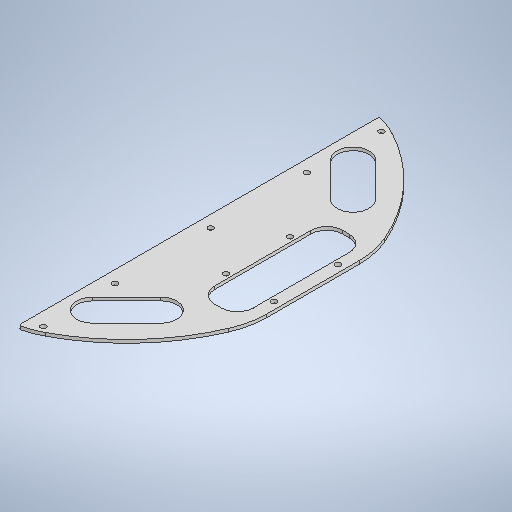
# Autodesk Inventor part: T2.0_frame-base2-extended-1
Saved by Autodesk Inventor 2025 (Build 290162000, 162)
## iProperties
Created: 2024-06-26
Part Number: T2.0_frame-base2-extended-1
Material: 一般
Document SubType Name: Sheet Metal
Designer: 8326d
Density: 1 g/cm^3
Sheet Metal Rule: Default_mm
Appearance: 既定
Author: 8326d
Autodesk Inventor part; units mm, degrees
ref_plane "YZ Plane" through (0, 0, 0) normal (1, 0, 0) x (0, 1, 0)
ref_plane "XZ Plane" through (0, 0, 0) normal (0, 1, 0) x (-1, 0, 0)
ref_plane "XY Plane" through (0, 0, 0) normal (0, 0, 1) x (1, 0, 0)
sketch "スケッチ1" plane through (0, 0, 0) normal (0, 1, 0) x (-1, 0, 0)
  circle A0 centre (0, 0) radius 122.5
  dimension "d0" = 245
  measures "d0" diameter of A0
extrude "プレート1" add sketch "スケッチ1" along normal blind 2
sketch "スケッチ2" plane through (0, 2, 0) normal (0, 1, 0) x (1, 0, 0)
  line L0 (85, -40) -> (109, -40)
  line L1 (109, -40) -> (109, 40)
  line L2 (109, 40) -> (85, 40)
  line L3 (85, 40) -> (85, -40)
  line L4 (85, -40) -> (109, 40) construction
  line L5 (109, -40) -> (85, 40) construction
  point P0 (0, 0)
  point P1 (97, 0)
  dimension "d2" = 24
  dimension "d3" = 85
  dimension "d6" = 80
  constraints: 12 end point, 2 midpoint, 2 parallel, 1 horizontal, 1 horizontal alignment, 1 perpendicular
  measures "d2" distance of L1.end L2.end
  measures "d3" distance from line of point (0, 0) L3
  measures "d6" distance of L0.end L1.end
extrude "押し出し1" cut sketch "スケッチ2" against normal through all
fillet "フィレット1" radius 10 4 edges at (109, 1, 40) (85, 1, 40) (85, 1, -40) (109, 1, -40)
sketch "スケッチ3" plane through (0, 2, 0) normal (0, 1, 0) x (1, 0, 0)
  line L0 (85, -30) -> (85, 30) projected
  line L1 (109, 30) -> (109, -30) projected
  line L2 (95, 40) -> (99, 40) projected
  line L3 (99, -40) -> (95, -40) projected
  line L4 (82, -20) -> (112, -20) construction
  line L5 (112, -20) -> (112, 20) construction
  line L6 (112, 20) -> (82, 20) construction
  line L7 (82, 20) -> (82, -20) construction
  line L8 (82, -20) -> (112, 20) construction
  line L9 (112, -20) -> (82, 20) construction
  point P0 (0, 0)
  point P1 (97, 0)
  point P2 (97, 40)
  point P3 (109, 0)
  dimension "d8" = 30
  dimension "d9" = 40
  constraints: 12 end point, 4 midpoint, 2 parallel, 1 horizontal, 1 horizontal alignment, 1 perpendicular, 1 vertical alignment
  measures "d8" distance of L6.end L5.end
  measures "d9" distance of L5.end L4.end
hole "穴1" at (82, 2, 20) at (112, 2, 20) at (112, 2, -20) at (82, 2, -20) direction (0, -1, 0) diameter 3.5 depth 2 tip angle 118
sketch "スケッチ4" plane through (0, 2, 0) normal (0, 1, 0) x (1, 0, 0)
  circle A0 centre (0, 0) radius 122.5 projected
  line L0 (-109.4589, 55) -> (-60, 30)
  line L1 (-60, 30) -> (-60, -30)
  line L2 (-60, -30) -> (-109.4589, -55)
  point P0 (-60, 0)
  dimension "d17" = 30
  dimension "d18" = 55
  dimension "d19" = 60
  constraints: 6 end point, 2 point on circle, 1 horizontal alignment, 1 midpoint, 1 vertical, 1 vertical alignment
  measures "d17" vertical distance of L1.end point (0, 0)
  measures "d18" vertical distance of point (0, 0) L0.start
  measures "d19" distance from line of point (0, 0) L1
extrude "押し出し2" cut sketch "スケッチ4" against normal through all contours L0 L1 L2 A0 picked at (-80.8333, 0)
sketch "スケッチ5" plane through (0, 2, 0) normal (0, 1, 0) x (1, 0, 0)
  line L0 (-40, 87) -> (40, 87)
  line L1 (40, 87) -> (40, 106)
  line L2 (40, 106) -> (-40, 106)
  line L3 (-40, 106) -> (-40, 87)
  line L4 (-40, 87) -> (40, 106) construction
  line L5 (40, 87) -> (-40, 106) construction
  line L6 (-13.5, 81.5) -> (13.5, 81.5)
  line L7 (13.5, 81.5) -> (13.5, 87)
  line L8 (13.5, 87) -> (-13.5, 87)
  line L9 (-13.5, 87) -> (-13.5, 81.5)
  line L10 (-13.5, 81.5) -> (13.5, 87) construction
  line L11 (13.5, 81.5) -> (-13.5, 87) construction
  line L12 (-13.5, 81.5) -> (-12.7575, 82.2425) construction
  line L13 (-13.5, 81.5) -> (-12.45, 81.5) construction
  line L14 (13.5, 81.5) -> (12.7575, 82.2425) construction
  line L15 (13.5, 81.5) -> (14.55, 81.5) construction
  circle A0 centre (12.7575, 82.2425) radius 1.05
  circle A1 centre (-12.7575, 82.2425) radius 1.05
  line L16 (-13.5, 111.5) -> (13.5, 111.5)
  line L17 (13.5, 111.5) -> (13.5, 106)
  line L18 (13.5, 106) -> (-13.5, 106)
  line L19 (-13.5, 106) -> (-13.5, 111.5)
  line L20 (-13.5, 111.5) -> (13.5, 106) construction
  line L21 (13.5, 111.5) -> (-13.5, 106) construction
  line L22 (-13.5, 111.5) -> (-12.7575, 110.7575) construction
  line L23 (-13.5, 111.5) -> (-12.45, 111.5) construction
  line L24 (13.5, 111.5) -> (12.7575, 110.7575) construction
  line L25 (13.5, 111.5) -> (14.55, 111.5) construction
  circle A2 centre (-12.7575, 110.7575) radius 1.05
  circle A3 centre (12.7575, 110.7575) radius 1.05
  point P0 (0, 0)
  point P1 (0, 96.5)
  point P2 (0, 84.25)
  point P3 (-13.5, 82.9849)
  point P4 (-12.0151, 81.5)
  point P5 (12.0151, 81.5)
  point P6 (13.5, 82.9849)
  point P7 (0, 108.75)
  point P8 (-13.5, 110.0151)
  point P9 (13.5, 110.0151)
  point P10 (12.0151, 111.5)
  point P11 (-12.0151, 111.5)
  dimension "d22" = 19
  dimension "d23" = 80
  dimension "d24" = 87
  dimension "d25" = 5.5
  dimension "d26" = 27
  dimension "d27" = 1.05
  dimension "d28" = 45
  dimension "d29" = 1.05
  dimension "d30" = 135
  dimension "d46" = 5.5
  dimension "d47" = 1.05
  dimension "d48" = 45
  dimension "d49" = 1.05
  dimension "d50" = 135
  constraints: 52 end point, 7 horizontal, 6 midpoint, 6 parallel, 4 coincident, 4 equal length, 4 vertical alignment, 3 perpendicular, 2 point on line, 12 other
  measures "d22" distance of L0.end L1.end
  measures "d23" distance of L1.end L2.end
  measures "d24" distance from line of point (0, 0) L0
  measures "d25" distance of L6.end L7.end
  measures "d26" distance of L6.start L6.end
  measures "d27" distance of L6.start L12.end
  measures "d28" angle of L13 L12
  measures "d29" distance of L6.end L14.end
  measures "d30" angle of L15 L14
  measures "d46" distance between parallel lines of L2 L16
  measures "d47" distance of L16.start L22.end
  measures "d48" angle of L22 L23
  measures "d49" distance of L16.end L24.end
  measures "d50" angle of L24 L25
extrude "押し出し3" cut sketch "スケッチ5" against normal through all
sketch "スケッチ6" plane through (0, 2, 0) normal (0, 1, 0) x (1, 0, 0)
  line L0 (-20, 84) -> (20, 84) construction
  line L1 (-20, 84) -> (20, 84) construction
  line L2 (12.0151, 81.5) -> (-12.0151, 81.5) construction
  line L3 (-20, 109) -> (20, 109) construction
  line L4 (13.5, 106) -> (40, 106) construction
  line L5 (-20, 109) -> (20, 109) construction
  line L6 (-12.0151, 111.5) -> (12.0151, 111.5) construction
  point P0 (0, 0)
  point P1 (0, 84)
  point P2 (0, 109)
  point P3 (0, 84)
  dimension "d33" = 40
  dimension "d34" = 0
  dimension "d35" = 2.5
  dimension "d51" = 40
  dimension "d52" = 0
  dimension "d53" = 2.5
  constraints: 8 end point, 3 horizontal, 3 midpoint, 2 collinear, 2 vertical alignment, 1 parallel
  measures "d33" distance of L0.start L0.end
  measures "d34" distance between parallel lines of L0 L1
  measures "d35" distance between parallel lines of L0 L2
  measures "d51" distance of L3.start L3.end
  measures "d52" distance between parallel lines of L3 L5
  measures "d53" distance between parallel lines of L6 L3
hole "穴2" at (20, 2, -84) at (-20, 2, -84) at (-20, 2, -109) at (20, 2, -109) direction (0, -1, 0) diameter 3.5 depth 2 tip angle 118
fillet "フィレット2" radius 1 4 edges at (-13.5, 1, -87) (13.5, 1, -87) (-13.5, 1, -106) (13.5, 1, -106)
fillet "フィレット3" radius 3 4 edges at (-40, 1, -87) (-40, 1, -106) (40, 1, -106) (40, 1, -87)
mirror "ミラー1" about plane through (0, 0, 0) normal (0, 0, 1) of "穴2", "押し出し3", "フィレット2", "フィレット3"
sketch "スケッチ8" plane through (0, 2, 0) normal (0, 1, 0) x (1, 0, 0)
  arc A0 (-109.4589, -55) -> (-109.4589, 55) centre (0, 0) ccw projected
  line L0 (-12.0151, 111.5) -> (12.0151, 111.5) projected
  line L1 (-44.8358, 114) -> (44.8358, 114)
  line L2 (-44.8358, -114) -> (44.8358, -114)
  line L3 (116.5, -37.8682) -> (116.5, 37.8682)
  arc A1 (-109.4589, -55) -> (-109.4589, 55) centre (0, 0) ccw projected
  circle A2 centre (112, 20) radius 1.75 projected
  line L4 (12.0151, -111.5) -> (-12.0151, -111.5) projected
  dimension "d61" = 4.5
  dimension "d62" = 2.5
  dimension "d63" = 2.5
  constraints: 6 end point, 6 point on circle, 1 horizontal, 1 parallel, 1 vertical
  measures "d61" distance from line of L3 A2.centre
  measures "d62" distance between parallel lines of L2 L4
  measures "d63" distance between parallel lines of L0 L1
extrude "押し出し5" cut sketch "スケッチ8" against normal through all contours L2 A0 | L3 A0 | L1 A0
fillet "フィレット5" radius 50 6 edges at (44.8358, 1, 114) (-44.8358, 1, 114) (116.5, 1, -37.8682) (116.5, 1, 37.8682) (-44.8358, 1, -114) (44.8358, 1, -114)
sketch "スケッチ9" plane through (0, 2, 0) normal (0, 1, 0) x (1, 0, 0)
  line L0 (12.0151, 81.5) -> (-12.0151, 81.5) projected
  line L1 (-14.5, 87) -> (-37, 87) projected
  line L2 (37, 87) -> (14.5, 87) projected
  point P0 (0, 0)
  point P1 (-35, 82)
  point P2 (-35, 74)
  point P3 (35, 82)
  point P4 (35, 74)
  dimension "d73" = 8
  dimension "d74" = 8
  dimension "d75" = 35
  dimension "d76" = 35
  dimension "d86" = 5
  dimension "d87" = 5
  constraints: 2 vertical alignment
  measures "d73" distance of point (-35, 74) point (-35, 82)
  measures "d74" distance of point (35, 74) point (35, 82)
  measures "d75" horizontal distance of point (0, 0) point (35, 82)
  measures "d76" horizontal distance of point (0, 0) point (-35, 82)
  measures "d86" distance from line of L1 point (-35, 82)
  measures "d87" distance from line of L2 point (35, 82)
hole "穴3" at (-35, 2, -82) at (-35, 2, -74) at (35, 2, -82) at (35, 2, -74) direction (0, -1, 0) diameter 3.2 end through all
sketch "スケッチ10" plane through (0, 2, 0) normal (0, 1, 0) x (1, 0, 0)
  line L0 (60.1041, 81.3173) -> (81.3173, 60.1041) construction
  line L1 (53.033, 74.2462) -> (74.2462, 53.033)
  line L2 (88.3883, 67.1751) -> (67.1751, 88.3883)
  arc A0 (67.1751, 88.3883) -> (53.033, 74.2462) centre (60.1041, 81.3173) ccw
  arc A1 (74.2462, 53.033) -> (88.3883, 67.1751) centre (81.3173, 60.1041) ccw
  line L3 (-15, 35) -> (15, 35) construction
  line L4 (-15, 20) -> (15, 20)
  line L5 (15, 50) -> (-15, 50)
  arc A2 (-15, 50) -> (-15, 20) centre (-15, 35) ccw
  arc A3 (15, 20) -> (15, 50) centre (15, 35) ccw
  line L6 (116.5, -28.8791) -> (116.5, 28.8791) projected
  line L7 (0, 0) -> (70.7107, 70.7107) construction
  point P0 (0, 35)
  dimension "d88" = 30
  dimension "d89" = 10
  dimension "d90" = 135
  dimension "d91" = 100
  dimension "d92" = 30
  dimension "d93" = 15
  dimension "d94" = 35
  constraints: 18 end point, 8 point on circle, 8 tangent, 4 centre point, 3 midpoint, 2 parallel, 1 horizontal, 1 perpendicular, 1 point on line, 1 vertical alignment
  measures "d88" distance of L0.start L0.end
  measures "d89" radius of A1
  measures "d90" angle of L6 L0
  measures "d91" distance of L7.start point (70.711, 70.711)
  measures "d92" distance of L3.start L3.end
  measures "d93" radius of A2
  measures "d94" distance from line of L7.start L3
extrude "押し出し6" cut sketch "スケッチ10" against normal through all
mirror "ミラー2" about plane through (0, 0, 0) normal (0, 0, 1) of "穴3", "押し出し6"
fillet "フィレット6" radius 2 4 edges at (-109.4589, 1, -55) (-60, 1, -30) (-60, 1, 30) (-109.4589, 1, 55)
sketch "スケッチ11" plane through (0, 2, 0) normal (0, 1, 0) x (1, 0, 0)
  arc A0 (-57.5538, 108.1379) -> (-108.5332, 56.8048) centre (0, 0) ccw projected
  arc A1 (-55.9094, 105.0483) -> (-106.3353, 53.4211) centre (0, 0) ccw construction
  line L0 (-107.6635, 54.0925) -> (-61.0978, 30.5549) construction
  line L1 (-106.3353, 53.4211) -> (0, 0) construction
  line L2 (0, 0) -> (-73.7957, 93.3552) construction
  point P0 (-103.9973, 57.8408)
  point P1 (-77.6522, 90.1728)
  dimension "d98" = 3.5
  dimension "d99" = 25
  dimension "d100" = 5
  dimension "d101" = 5
  constraints: 5 point on circle, 4 end point, 1 centre point, 1 point on line
  measures "d98" radial gap between concentric circles of A0 A1
  measures "d99" angle of L1 L2
  measures "d100" distance of L2.end point (-77.652, 90.173)
  measures "d101" distance of L1.start point (-103.997, 57.841)
hole "穴4" at (-103.9973, 2, -57.8408) at (-77.6522, 2, -90.1728) direction (0, -1, 0) diameter 3.5 end through all
mirror "ミラー3" about plane through (0, 0, 0) normal (0, 0, 1) of "穴4"
sketch "スケッチ12" plane through (0, 2, 0) normal (0, 1, 0) x (1, 0, 0)
  line L0 (-52, 45) -> (-52, 35) construction
  line L1 (-52, 45) -> (-42, 45) construction
  line L2 (-52, -35) -> (-52, -45) construction
  line L3 (-52, -35) -> (-42, -35) construction
  point P0 (0, 0)
  point P1 (-52, 40)
  point P2 (-52, -40)
  dimension "d109" = 10
  dimension "d110" = 90
  dimension "d111" = 10
  dimension "d112" = 90
  dimension "d113" = 40
  dimension "d114" = 40
  dimension "d115" = 52
  dimension "d116" = 52
  constraints: 8 end point, 4 coincident, 2 horizontal, 2 midpoint, 2 perpendicular, 2 vertical
  measures "d109" distance of L0.start L0.end
  measures "d110" angle of L0 L1
  measures "d111" distance of L2.start L2.end
  measures "d112" angle of L2 L3
  measures "d113" vertical distance of point (0, 0) point (-52, 40)
  measures "d114" vertical distance of point (0, 0) point (-52, -40)
  measures "d115" distance from line of point (0, 0) L0
  measures "d116" distance from line of point (0, 0) L2
hole "穴5" at (-52, 2, -45) at (-52, 2, -35) at (-52, 2, 35) at (-52, 2, 45) direction (0, -1, 0) diameter 3.5 depth 2
sketch "スケッチ13" plane through (0, 2, 0) normal (0, 1, 0) x (1, 0, 0)
  arc A0 (57.5538, 108.1379) -> (34.0624, 114) centre (34.0624, 64) ccw projected
  arc A1 (34.0624, -114) -> (57.5538, -108.1379) centre (34.0624, -64) ccw projected
  line L0 (45, 112.789) -> (45, -112.789) construction
  line L1 (45, 112.789) -> (270.5781, 112.789) construction
  line L2 (37.5, -60) -> (52.5, -60) construction
  line L3 (52.5, -60) -> (52.5, 60) construction
  line L4 (52.5, 60) -> (37.5, 60) construction
  line L5 (37.5, 60) -> (37.5, -60) construction
  line L6 (37.5, -60) -> (52.5, 60) construction
  line L7 (52.5, -60) -> (37.5, 60) construction
  arc A2 (34.0624, -110) -> (53.5029, -105.6902) centre (34.0624, -64) ccw construction
  line L8 (34.0624, -64) -> (53.5029, -105.6902) construction
  line L9 (34.0624, -64) -> (34.0624, -110) construction
  arc A3 (53.5029, 105.6902) -> (34.0624, 110) centre (34.0624, 64) ccw construction
  line L10 (34.0624, 64) -> (34.0624, 110) construction
  line L11 (34.0624, 64) -> (80.0624, 64) construction
  line L12 (34.0624, 64) -> (53.5029, 105.6902) construction
  point P0 (0, 0)
  point P1 (45, 0)
  point P2 (52.5, 0)
  point P3 (37.5, 0)
  dimension "d124" = 90
  dimension "d125" = 45
  dimension "d126" = 15
  dimension "d127" = 120
  dimension "d135" = 25
  dimension "d136" = 46
  dimension "d137" = 46
  dimension "d138" = 90
  dimension "d139" = 25
  constraints: 26 end point, 10 coincident, 6 point on circle, 5 midpoint, 3 horizontal, 3 perpendicular, 2 centre point, 2 parallel, 1 vertical alignment
  measures "d124" angle of L0 L1
  measures "d125" distance from line of point (0, 0) L0
  measures "d126" distance of L4.end L3.end
  measures "d127" distance of L3.end L2.end
  measures "d135" angle of L9 L8
  measures "d136" radius of A2
  measures "d137" radius of A3
  measures "d138" angle of L11 L10
  measures "d139" angle of L12 L10
hole "穴6" at (37.5, 2, -60) at (52.5, 2, -60) at (52.5, 2, 0) at (37.5, 2, 0) at (37.5, 2, 60) at (52.5, 2, 60) at (34.0624, 2, -110) at (53.5029, 2, -105.6902) at (34.0624, 2, 110) at (53.5029, 2, 105.6902) direction (0, -1, 0) diameter 3.5 end through all
sketch "スケッチ14" plane through (0, 2, 0) normal (0, 1, 0) x (1, 0, 0)
  arc A0 (57.5538, 108.1379) -> (34.0624, 114) centre (34.0624, 64) ccw projected
  line L0 (34.0624, 114) -> (-34.0624, 114) projected
  arc A1 (-34.0624, 114) -> (-57.5538, 108.1379) centre (-34.0624, 64) ccw projected
  arc A2 (-57.5538, 108.1379) -> (-108.5332, 56.8048) centre (0, 0) ccw projected
  arc A3 (-108.5332, 56.8048) -> (-107.6635, 54.0925) centre (-106.7613, 55.8774) ccw projected
  line L1 (-107.6635, 54.0925) -> (-61.0978, 30.5549) projected
  arc A4 (-60, 28.77) -> (-61.0978, 30.5549) centre (-62, 28.77) ccw projected
  line L2 (-60, 28.77) -> (-60, -28.77) projected
  arc A5 (-61.0978, -30.5549) -> (-60, -28.77) centre (-62, -28.77) ccw projected
  line L3 (-61.0978, -30.5549) -> (-107.6635, -54.0925) projected
  arc A6 (-107.6635, -54.0925) -> (-108.5332, -56.8048) centre (-106.7613, -55.8774) ccw projected
  arc A7 (-108.5332, -56.8048) -> (-57.5538, -108.1379) centre (0, 0) ccw projected
  arc A8 (-57.5538, -108.1379) -> (-34.0624, -114) centre (-34.0624, -64) ccw projected
  line L4 (-34.0624, -114) -> (34.0624, -114) projected
  arc A9 (34.0624, -114) -> (57.5538, -108.1379) centre (34.0624, -64) ccw projected
  line L5 (45, -112.789) -> (45, 112.789)
  arc A10 (57.5538, 108.1379) -> (34.0624, 114) centre (34.0624, 64) ccw projected
  dimension "d140" = 45
  constraints: 2 end point, 2 point on circle, 1 vertical
  measures "d140" distance from line of L5 point (0, 0)
extrude "押し出し7" cut sketch "スケッチ14" against normal through all
fillet "フィレット7" radius 1 2 edges at (45, 1, 112.789) (45, 1, -112.789)
equation "\"d15\" = Thickness"
equation "\"d46\" = d25"
equation "\"d53\" = d35"
equation "\"d41\" = Thickness"
equation "\"d63\" = d62"
equation "\"d73\" = d71"
equation "\"d74\" = d71"
equation "\"d76\" = d75"
equation "\"d87\" = d86"
equation "\"d84\" = Thickness"
equation "\"d101\" = d100"
equation "\"d107\" = Thickness"
equation "\"d114\" = d113"
equation "\"d116\" = d115"
equation "\"d122\" = Thickness"
equation "\"d133\" = Thickness"
equation "\"d1\" = Thickness"
equation "\"BendRadius\" = Thickness"
equation "\"BendReliefWidth\" = Thickness"
equation "\"BendReliefDepth\" = 0.5 * Thickness"
equation "\"CornerReliefSize\" = 4 * Thickness"
equation "\"MinimumRemnant\" = 2 * Thickness"
equation "\"TransitionRadius\" = BendRadius"
equation "\"JacobiRadiusSize\" = BendRadius"
equation "\"GapSize\" = Thickness"
equation "\"Thickness\" = 2"
equation "\"d71\" = 8"
